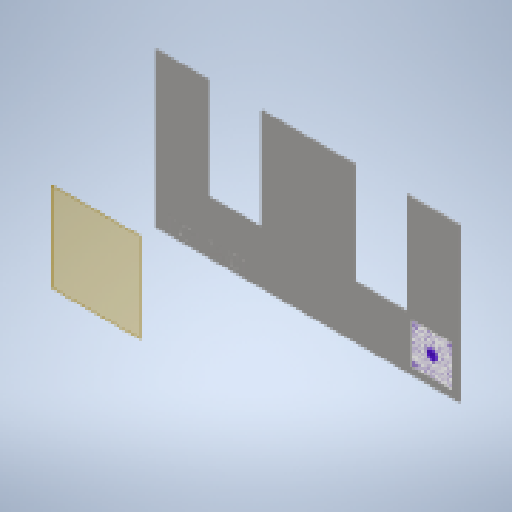
# Autodesk Inventor part: Chapa
Saved by Autodesk Inventor 2025 (Build 290162000, 162)
## iProperties
Created: 2024-05-06
Part Number: Chapa
Material: Steel, Alloy
Document SubType Name: Modeling
Designer: 082220019
Density: 7.73 g/cm^3
Appearance: Semi-Polished
Author: 082220019
Autodesk Inventor part; units mm, degrees
ref_plane "YZ Plane" through (0, 0, 0) normal (1, 0, 0) x (0, 1, 0)
ref_plane "XZ Plane" through (0, 0, 0) normal (0, 1, 0) x (-1, 0, 0)
ref_plane "XY Plane" through (0, 0, 0) normal (0, 0, 1) x (1, 0, 0)
sketch "Sketch1" plane through (0, 0, 0) normal (0, 0, 1) x (1, 0, 0)
  line L0 (0, 0) -> (0, 38)
  line L1 (0, 38) -> (13, 38)
  line L2 (13, 38) -> (13, 13)
  line L3 (13, 13) -> (26, 13)
  line L4 (26, 13) -> (26, 38)
  line L5 (26, 38) -> (49, 38)
  line L6 (49, 38) -> (49, 13)
  line L7 (49, 13) -> (62, 13)
  line L8 (62, 13) -> (62, 38)
  line L9 (62, 38) -> (75, 38)
  line L10 (75, 38) -> (75, 0)
  line L11 (75, 0) -> (0, 0)
  point P0 (19.5, 13)
  dimension "d0" = 23
  dimension "d1" = 13
  dimension "d2" = 13
  dimension "d3" = 38
  dimension "d4" = 75
  dimension "d5" = 13
  dimension "d6" = 13
  dimension "d7" = 13
  constraints: 24 end point, 6 point on line, 5 perpendicular, 2 parallel, 2 vertical, 1 collinear, 1 midpoint
  measures "d0" distance of L4.end L5.end
  measures "d1" distance of L0.end L1.end
  measures "d2" distance from line of L11 point (19.5, 13)
  measures "d3" distance of L9.end L10.end
  measures "d4" distance of L10.end L0.start
  measures "d5" distance of L4.end L1.end
  measures "d6" distance of L6.end L7.end
  measures "d7" distance of L8.end L9.end
extrude "Extrusion1" add sketch "Sketch1" along normal blind 0.3556
ref_plane "Work Plane2" through (0, 0, 15.1056) normal (0, 0, 1) x (1, 0, 0)
sketch "Sketch2" plane through (0, 0, 15.1056) normal (0, 0, 1) x (1, 0, 0)
  line L0 (2.7449, 4.3303) -> (27.4135, 4.3303) construction
  line L1 (27.4135, 4.3303) -> (27.4135, 0.8062) construction
  line L2 (27.4135, 0.8062) -> (2.7449, 0.8062) construction
  line L3 (2.7449, 0.8062) -> (2.7449, 4.3303) construction
  line L4 (3.7067, 4.0139) -> (3.7067, 2.8103)
  line L5 (3.7067, 2.8103) -> (4.377, 2.8103)
  spline S0 degree 2 poles (4.377, 2.8103) (4.6387, 2.8103) (4.7259, 2.89) knots 0 0 0 1 1 1
  spline S1 degree 2 poles (4.7259, 2.89) (4.8455, 2.9922) (4.8579, 3.2539) knots 0 0 0 1 1 1
  line L6 (4.8579, 3.2539) -> (4.9402, 3.2539)
  line L7 (4.9402, 3.2539) -> (4.9402, 2.1898)
  line L8 (4.9402, 2.1898) -> (4.8579, 2.1898)
  spline S2 degree 2 poles (4.8579, 2.1898) (4.8256, 2.4116) (4.7956, 2.4739) knots 0 0 0 1 1 1
  spline S3 degree 2 poles (4.7956, 2.4739) (4.7533, 2.5536) (4.5689, 2.6434) (4.377, 2.6434) knots 0 0 0 1 2 2 2
  line L9 (4.377, 2.6434) -> (3.7067, 2.6434)
  line L10 (3.7067, 2.6434) -> (3.7067, 1.6391)
  spline S4 degree 2 poles (3.7067, 1.6391) (3.7067, 1.4373) (3.7416, 1.3501) (3.8338, 1.2978) (3.9584, 1.2978) knots 0 0 0 1 2 3 3 3
  line L11 (3.9584, 1.2978) -> (4.4767, 1.2978)
  spline S5 degree 2 poles (4.4767, 1.2978) (4.7358, 1.2978) (4.9701, 1.37) (5.0772, 1.4747) knots 0 0 0 1 2 2 2
  spline S6 degree 2 poles (5.0772, 1.4747) (5.2168, 1.6142) (5.3638, 1.8958) knots 0 0 0 1 1 1
  line L12 (5.3638, 1.8958) -> (5.4535, 1.8958)
  line L13 (5.4535, 1.8958) -> (5.1894, 1.1308)
  line L14 (5.1894, 1.1308) -> (2.8396, 1.1308)
  line L15 (2.8396, 1.1308) -> (2.8396, 1.213)
  line L16 (2.8396, 1.213) -> (2.9467, 1.213)
  spline S7 degree 2 poles (2.9467, 1.213) (3.0564, 1.213) (3.151, 1.2654) knots 0 0 0 1 1 1
  spline S8 degree 2 poles (3.151, 1.2654) (3.2233, 1.3027) (3.2756, 1.4473) (3.2756, 1.6715) knots 0 0 0 1 2 2 2
  line L17 (3.2756, 1.6715) -> (3.2756, 3.6501)
  spline S9 degree 2 poles (3.2756, 3.6501) (3.2756, 3.9416) (3.2183, 4.0089) knots 0 0 0 1 1 1
  spline S10 degree 2 poles (3.2183, 4.0089) (3.1361, 4.0986) (2.9467, 4.0986) knots 0 0 0 1 1 1
  line L18 (2.9467, 4.0986) -> (2.8396, 4.0986)
  line L19 (2.8396, 4.0986) -> (2.8396, 4.1808)
  line L20 (2.8396, 4.1808) -> (5.1918, 4.1808)
  line L21 (5.1918, 4.1808) -> (5.2242, 3.5105)
  line L22 (5.2242, 3.5105) -> (5.137, 3.5105)
  spline S11 degree 2 poles (5.137, 3.5105) (5.0897, 3.7522) (4.9751, 3.9316) (4.8629, 3.979) knots 0 0 0 1 2 2 2
  spline S12 degree 2 poles (4.8629, 3.979) (4.7732, 4.0139) (4.544, 4.0139) knots 0 0 0 1 1 1
  line L23 (4.544, 4.0139) -> (3.7067, 4.0139)
  line L24 (8.3316, 4.2506) -> (8.4013, 3.214)
  line L25 (8.4013, 3.214) -> (8.3316, 3.214)
  spline S13 degree 2 poles (8.3316, 3.214) (8.192, 3.68) (7.6762, 4.0911) (7.3149, 4.0911) knots 0 0 0 1 2 2 2
  spline S14 degree 2 poles (7.3149, 4.0911) (7.0134, 4.0911) (6.525, 3.7821) (6.2434, 3.1068) (6.2434, 2.6035) knots 0 0 0 1 2 3 3 3
  spline S15 degree 2 poles (6.2434, 2.6035) (6.2434, 2.1898) (6.5075, 1.5818) (7.0408, 1.2579) (7.3797, 1.2579) knots 0 0 0 1 2 3 3 3
  spline S16 degree 2 poles (7.3797, 1.2579) (7.6762, 1.2579) (8.1297, 1.5121) (8.4013, 1.8908) knots 0 0 0 1 2 2 2
  line L26 (8.4013, 1.8908) -> (8.4711, 1.846)
  spline S17 degree 2 poles (8.4711, 1.846) (8.2418, 1.4398) (7.6314, 1.061) (7.2102, 1.061) knots 0 0 0 1 2 2 2
  spline S18 degree 2 poles (7.2102, 1.061) (6.4527, 1.061) (6.0366, 1.6242) knots 0 0 0 1 1 1
  spline S19 degree 2 poles (6.0366, 1.6242) (5.7276, 2.0428) (5.7276, 2.6085) knots 0 0 0 1 1 1
  spline S20 degree 2 poles (5.7276, 2.6085) (5.7276, 3.0645) (6.1363, 3.8295) (6.8539, 4.2506) (7.2775, 4.2506) knots 0 0 0 1 2 3 3 3
  spline S21 degree 2 poles (7.2775, 4.2506) (7.6064, 4.2506) (7.9279, 4.0886) knots 0 0 0 1 1 1
  spline S22 degree 2 poles (7.9279, 4.0886) (8.0226, 4.0388) (8.0624, 4.0388) knots 0 0 0 1 1 1
  spline S23 degree 2 poles (8.0624, 4.0388) (8.1247, 4.0388) (8.1696, 4.0811) knots 0 0 0 1 1 1
  spline S24 degree 2 poles (8.1696, 4.0811) (8.2269, 4.1434) (8.2518, 4.2506) knots 0 0 0 1 1 1
  line L27 (8.2518, 4.2506) -> (8.3316, 4.2506)
  line L28 (10.776, 2.2546) -> (10.776, 1.9357)
  line L29 (10.776, 1.9357) -> (10.3674, 1.9357)
  line L30 (10.3674, 1.9357) -> (10.3674, 1.1308)
  line L31 (10.3674, 1.1308) -> (9.9961, 1.1308)
  line L32 (9.9961, 1.1308) -> (9.9961, 1.9357)
  line L33 (9.9961, 1.9357) -> (8.7028, 1.9357)
  line L34 (8.7028, 1.9357) -> (8.7028, 2.2222)
  line L35 (8.7028, 2.2222) -> (10.1207, 4.2431)
  line L36 (10.1207, 4.2431) -> (10.3674, 4.2431)
  line L37 (10.3674, 4.2431) -> (10.3674, 2.2546)
  line L38 (10.3674, 2.2546) -> (10.776, 2.2546)
  line L39 (9.9961, 2.2546) -> (9.9961, 3.7697)
  line L40 (9.9961, 3.7697) -> (8.9246, 2.2546)
  line L41 (8.9246, 2.2546) -> (9.9961, 2.2546)
  line L42 (11.1224, 2.3344) -> (12.2886, 2.3344)
  line L43 (12.2886, 2.3344) -> (12.2886, 1.9955)
  line L44 (12.2886, 1.9955) -> (11.1224, 1.9955)
  line L45 (11.1224, 1.9955) -> (11.1224, 2.3344)
  line L46 (14.5836, 1.7164) -> (14.3693, 1.1308)
  line L47 (14.3693, 1.1308) -> (12.5702, 1.1308)
  line L48 (12.5702, 1.1308) -> (12.5702, 1.213)
  spline S25 degree 2 poles (12.5702, 1.213) (13.3651, 1.9382) (14.0129, 2.8552) (14.0129, 3.2364) knots 0 0 0 1 2 2 2
  spline S26 degree 2 poles (14.0129, 3.2364) (14.0129, 3.5255) (13.6566, 3.8992) (13.4099, 3.8992) knots 0 0 0 1 2 2 2
  spline S27 degree 2 poles (13.4099, 3.8992) (13.1831, 3.8992) (12.8268, 3.6351) (12.7396, 3.3809) knots 0 0 0 1 2 2 2
  line L49 (12.7396, 3.3809) -> (12.6574, 3.3809)
  spline S28 degree 2 poles (12.6574, 3.3809) (12.7147, 3.7971) (13.1782, 4.2431) (13.527, 4.2431) knots 0 0 0 1 2 2 2
  spline S29 degree 2 poles (13.527, 4.2431) (13.8983, 4.2431) (14.3967, 3.7672) (14.3967, 3.4432) knots 0 0 0 1 2 2 2
  spline S30 degree 2 poles (14.3967, 3.4432) (14.3967, 3.2115) (14.2895, 2.9797) knots 0 0 0 1 1 1
  spline S31 degree 2 poles (14.2895, 2.9797) (14.1226, 2.6159) (13.7488, 2.2073) knots 0 0 0 1 1 1
  spline S32 degree 2 poles (13.7488, 2.2073) (13.1881, 1.5968) (13.0486, 1.4697) knots 0 0 0 1 1 1
  line L50 (13.0486, 1.4697) -> (13.846, 1.4697)
  spline S33 degree 2 poles (13.846, 1.4697) (14.0902, 1.4697) (14.2845, 1.5046) (14.4415, 1.6167) (14.5013, 1.7164) knots 0 0 0 1 2 3 3 3
  line L51 (14.5013, 1.7164) -> (14.5836, 1.7164)
  line L52 (16.9209, 2.2546) -> (16.9209, 1.9357)
  line L53 (16.9209, 1.9357) -> (16.5122, 1.9357)
  line L54 (16.5122, 1.9357) -> (16.5122, 1.1308)
  line L55 (16.5122, 1.1308) -> (16.141, 1.1308)
  line L56 (16.141, 1.1308) -> (16.141, 1.9357)
  line L57 (16.141, 1.9357) -> (14.8477, 1.9357)
  line L58 (14.8477, 1.9357) -> (14.8477, 2.2222)
  line L59 (14.8477, 2.2222) -> (16.2655, 4.2431)
  line L60 (16.2655, 4.2431) -> (16.5122, 4.2431)
  line L61 (16.5122, 4.2431) -> (16.5122, 2.2546)
  line L62 (16.5122, 2.2546) -> (16.9209, 2.2546)
  line L63 (16.141, 2.2546) -> (16.141, 3.7697)
  line L64 (16.141, 3.7697) -> (15.0695, 2.2546)
  line L65 (15.0695, 2.2546) -> (16.141, 2.2546)
  line L66 (18.3686, 4.3303) -> (17.2648, 1.0685)
  line L67 (17.2648, 1.0685) -> (17.0854, 1.0685)
  line L68 (17.0854, 1.0685) -> (18.1892, 4.3303)
  line L69 (18.1892, 4.3303) -> (18.3686, 4.3303)
  spline S34 degree 2 poles (18.5281, 2.6384) (18.5281, 3.1592) (18.8421, 3.9117) (19.1037, 4.0961) knots 0 0 0 1 2 2 2
  spline S35 degree 2 poles (19.1037, 4.0961) (19.3056, 4.2431) (19.5224, 4.2431) knots 0 0 0 1 1 1
  spline S36 degree 2 poles (19.5224, 4.2431) (19.8737, 4.2431) (20.1528, 3.8868) knots 0 0 0 1 1 1
  spline S37 degree 2 poles (20.1528, 3.8868) (20.5017, 3.4432) (20.5017, 2.6857) knots 0 0 0 1 1 1
  spline S38 degree 2 poles (20.5017, 2.6857) (20.5017, 2.155) (20.1952, 1.4124) (19.7217, 1.0785) (19.4999, 1.0785) knots 0 0 0 1 2 3 3 3
  spline S39 degree 2 poles (19.4999, 1.0785) (19.0639, 1.0785) (18.7723, 1.5943) knots 0 0 0 1 1 1
  spline S40 degree 2 poles (18.7723, 1.5943) (18.5281, 2.0279) (18.5281, 2.6384) knots 0 0 0 1 1 1
  spline S41 degree 2 poles (18.9692, 2.5811) (18.9692, 1.9531) (19.1237, 1.5544) knots 0 0 0 1 1 1
  spline S42 degree 2 poles (19.1237, 1.5544) (19.2532, 1.2205) (19.5074, 1.2205) knots 0 0 0 1 1 1
  spline S43 degree 2 poles (19.5074, 1.2205) (19.6295, 1.2205) (19.8887, 1.4373) (19.9559, 1.694) knots 0 0 0 1 2 2 2
  spline S44 degree 2 poles (19.9559, 1.694) (20.0606, 2.0802) (20.0606, 2.7829) knots 0 0 0 1 1 1
  spline S45 degree 2 poles (20.0606, 2.7829) (20.0606, 3.3062) (19.9535, 3.6525) knots 0 0 0 1 1 1
  spline S46 degree 2 poles (19.9535, 3.6525) (19.8712, 3.9117) (19.7441, 4.0188) knots 0 0 0 1 1 1
  spline S47 degree 2 poles (19.7441, 4.0188) (19.6519, 4.0936) (19.5199, 4.0936) knots 0 0 0 1 1 1
  spline S48 degree 2 poles (19.5199, 4.0936) (19.3679, 4.0936) (19.2483, 3.9565) knots 0 0 0 1 1 1
  spline S49 degree 2 poles (19.2483, 3.9565) (19.0863, 3.7697) (18.9692, 2.9698) (18.9692, 2.5811) knots 0 0 0 1 2 2 2
  line L70 (21.2043, 3.8818) -> (21.9469, 4.2431)
  line L71 (21.9469, 4.2431) -> (22.0217, 4.2431)
  line L72 (22.0217, 4.2431) -> (22.0217, 1.669)
  spline S50 degree 2 poles (22.0217, 1.669) (22.0217, 1.4124) (22.064, 1.2853) (22.1986, 1.218) (22.4054, 1.213) knots 0 0 0 1 2 3 3 3
  line L73 (22.4054, 1.213) -> (22.4054, 1.1308)
  line L74 (22.4054, 1.1308) -> (21.2592, 1.1308)
  line L75 (21.2592, 1.1308) -> (21.2592, 1.213)
  spline S51 degree 2 poles (21.2592, 1.213) (21.476, 1.218) (21.6006, 1.2828) (21.6504, 1.3925) (21.6504, 1.669) knots 0 0 0 1 2 3 3 3
  line L76 (21.6504, 1.669) -> (21.6504, 3.3137)
  spline S52 degree 2 poles (21.6504, 3.3137) (21.6504, 3.6476) (21.628, 3.7422) knots 0 0 0 1 1 1
  spline S53 degree 2 poles (21.628, 3.7422) (21.613, 3.8145) (21.5283, 3.8818) (21.471, 3.8818) knots 0 0 0 1 2 2 2
  spline S54 degree 2 poles (21.471, 3.8818) (21.3863, 3.8818) (21.2392, 3.812) knots 0 0 0 1 1 1
  line L77 (21.2392, 3.812) -> (21.2043, 3.8818)
  point P0 (0, 0)
  constraints: 2 other
emboss "Emboss1" sketch "Sketch2" operation cut depth 0.3 direction (0, 0, -1)
ref_plane "Work Plane3" through (0, 0, 15.1056) normal (0, 0, 1) x (1, 0, 0)
sketch "Sketch3" plane through (0, 0, 15.1056) normal (0, 0, 1) x (1, 0, 0)
  line L0 (63.3018, 11.8743) -> (73.3018, 11.8743) construction
  line L1 (73.3018, 11.8743) -> (73.3018, 1.8743) construction
  line L2 (73.3018, 1.8743) -> (63.3018, 1.8743) construction
  line L3 (63.3018, 1.8743) -> (63.3018, 11.8743) construction
  point P0 (0, 0)
  dimension "d14" = 10
  constraints: 2 other
  measures "d14" distance of L0.start L0.end
decal "Decal1"
body "Solid1"
